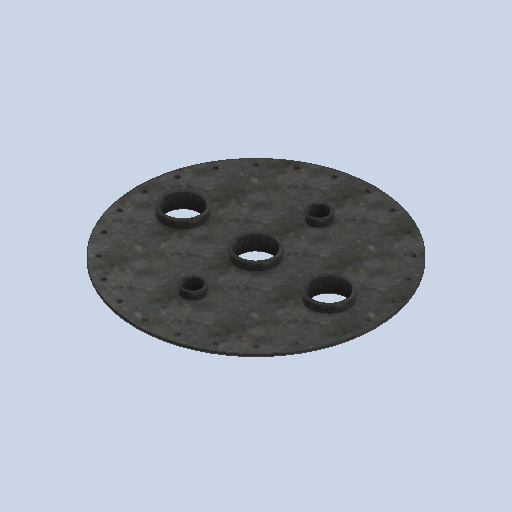
# Autodesk Inventor part: Tapa2
Saved by Autodesk Inventor 2023 (Build 270158000, 158)
## iProperties
Created: 2022-11-02
Part Number: Tapa2
Material: Steel ASTM A36
Document SubType Name: Modeling
Designer: Juanse
Density: 7.85 g/cm^3
Appearance: Plate
Author: Juanse
Autodesk Inventor part; units mm, degrees
ref_plane "YZ Plane" through (0, 0, 0) normal (1, 0, 0) x (0, 1, 0)
ref_plane "XZ Plane" through (0, 0, 0) normal (0, 1, 0) x (-1, 0, 0)
ref_plane "XY Plane" through (0, 0, 0) normal (0, 0, 1) x (1, 0, 0)
sketch "Sketch1" plane through (0, 0, 0) normal (0, 1, 0) x (-1, 0, 0)
  circle A0 centre (0, 0) radius 360
  circle A1 centre (0, 0) radius 335 construction
  circle A2 centre (335, 0) radius 7.1437
  circle A3 centre (0, 0) radius 50.8
  circle A4 centre (220, 0) radius 50.8
  circle A5 centre (-220, 0) radius 50.8
  circle A6 centre (0, -190) radius 25.4
  circle A7 centre (0, 190) radius 25.4
  circle A8 centre (0, 0) radius 190 construction
  circle A9 centre (0, 0) radius 220 construction
  dimension "d1" = 670
  dimension "d0" = 720
  dimension "d2" = 14.2875
  dimension "d3" = 101.6
  dimension "d4" = 101.6
  dimension "d5" = 101.6
  dimension "d6" = 50.8
  dimension "d7" = 50.8
  dimension "d8" = 380
  dimension "d23" = 440
  constraints: 9 centre point, 5 coincident, 4 horizontal alignment, 4 point on circle, 2 vertical alignment, 2 other
  measures "d0" diameter of A0
  measures "d2" diameter of A2
  measures "d3" diameter of A3
  measures "d4" diameter of A5
  measures "d5" diameter of A4
  measures "d6" diameter of A6
  measures "d7" diameter of A7
  measures "d8" diameter of A8
  measures "d23" diameter of A9
extrude "Extrusion1" add sketch "Sketch1" along normal blind 8 contours A0 | A2
extrude "Extrusion2" cut sketch "Sketch1" along normal through all contours A2
pattern_circular "Circular Pattern1" count 24 over 360 about axis through (0, 0, 0) along (0, 1, 0) of "Extrusion2"
sketch "Sketch2" plane through (0, 8, 0) normal (0, 1, 0) x (1, 0, 0)
  circle A0 centre (-323.5852, 86.7044) radius 7.1437 projected
  circle A1 centre (-290.1185, 167.5) radius 7.1437 projected
  circle A2 centre (-236.8808, 236.8808) radius 7.1437 projected
  circle A3 centre (-167.5, 290.1185) radius 7.1437 projected
  circle A4 centre (-86.7044, 323.5852) radius 7.1437 projected
  circle A5 centre (0, 335) radius 7.1437 projected
  circle A6 centre (86.7044, 323.5852) radius 7.1437 projected
  circle A7 centre (167.5, 290.1185) radius 7.1437 projected
  circle A8 centre (236.8808, 236.8808) radius 7.1437 projected
  circle A9 centre (290.1185, 167.5) radius 7.1437 projected
  circle A10 centre (323.5852, 86.7044) radius 7.1437 projected
  circle A11 centre (335, 0) radius 7.1437 projected
  circle A12 centre (323.5852, -86.7044) radius 7.1437 projected
  circle A13 centre (290.1185, -167.5) radius 7.1437 projected
  circle A14 centre (236.8808, -236.8808) radius 7.1437 projected
  circle A15 centre (167.5, -290.1185) radius 7.1437 projected
  circle A16 centre (86.7044, -323.5852) radius 7.1437 projected
  circle A17 centre (0, -335) radius 7.1437 projected
  circle A18 centre (-86.7044, -323.5852) radius 7.1437 projected
  circle A19 centre (-167.5, -290.1185) radius 7.1437 projected
  circle A20 centre (-236.8808, -236.8808) radius 7.1437 projected
  circle A21 centre (-290.1185, -167.5) radius 7.1437 projected
  circle A22 centre (-323.5852, -86.7044) radius 7.1437 projected
  circle A23 centre (-335, 0) radius 7.1437 projected
  circle A24 centre (0, 0) radius 360 projected
  circle A25 centre (0, 0) radius 50.8 projected
  circle A26 centre (-220, 0) radius 50.8 projected
  circle A27 centre (220, 0) radius 50.8 projected
  circle A28 centre (0, 190) radius 25.4 projected
  circle A29 centre (0, -190) radius 25.4 projected
  circle A30 centre (0, 190) radius 25.4 projected
  circle A31 centre (0, 190) radius 31.4
  circle A32 centre (220, 0) radius 50.8 projected
  circle A33 centre (220, 0) radius 58.8
  circle A34 centre (0, 0) radius 58.8
  circle A35 centre (0, -190) radius 31.4
  circle A36 centre (-220, 0) radius 58.8
  dimension "d16" = 6
  dimension "d17" = 8
  dimension "d18" = 8
  dimension "d19" = 8
  dimension "d20" = 6
  constraints: 5 centre point, 5 coincident
  measures "d16" radial gap between concentric circles of A28 A31
  measures "d17" radial gap between concentric circles of A34 A25
  measures "d18" radial gap between concentric circles of A27 A33
  measures "d19" radial gap between concentric circles of A26 A36
  measures "d20" radial gap between concentric circles of A35 A29
extrude "Extrusion3" add sketch "Sketch2" along normal mid plane 45 contours A31 | A33 | A34 | A35 | A36
equation "\"d4\" = d3"
equation "\"d5\" = d3"
equation "\"d6\" = 0.5 * d3"
equation "\"d7\" = 0.5 * d3"
equation "\"d18\" = d17"
equation "\"d19\" = d17"
equation "\"d20\" = d16"
body "Solid1"
